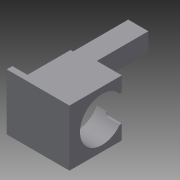
# Autodesk Inventor part: BF_base_model
Saved by Autodesk Inventor 2015 SP2 (Build 190223200, 223)
## iProperties
Created: 2016-08-30
Part Number: BF_base_model
Material: Generic
Document SubType Name: Modeling
Designer: jm799
Density: 1 g/cm^3
Appearance: Default
Author: jm799
Autodesk Inventor part; units mm, degrees
ref_plane "YZ Plane" through (0, 0, 0) normal (1, 0, 0) x (0, 1, 0)
ref_plane "XZ Plane" through (0, 0, 0) normal (0, 1, 0) x (-1, 0, 0)
ref_plane "XY Plane" through (0, 0, 0) normal (0, 0, 1) x (1, 0, 0)
sketch "Sketch1" plane through (0, 0, 0) normal (0, 1, 0) x (-1, 0, 0)
  line L0 (16.2222, 35.2121) -> (-14.7778, 35.2121)
  line L1 (-14.7778, 35.2121) -> (-14.7778, -34.7879)
  line L2 (-14.7778, -34.7879) -> (16.2222, -34.7879)
  line L3 (16.2222, -34.7879) -> (16.2222, 35.2121)
  point P0 (0, 0)
  dimension "d0" = 70
  dimension "d1" = 31
  constraints: 8 end point, 2 parallel, 1 horizontal, 1 perpendicular
  measures "d0" distance of L0.end L1.end
  measures "d1" distance of L0.start L0.end
extrude "Extrusion1" add sketch "Sketch1" along normal blind 60
sketch "Sketch3" plane through (14.7778, 0, 35.2121) normal (1, 0, 0) x (0, 0, -1)
  circle A0 centre (35.2121, 35.5368) radius 27.5
  point P0 (35.2121, 0)
  dimension "d5" = 55
  constraints: 1 centre point
  measures "d5" diameter of A0
hole "Hole1" at (14.7778, 35.5368, 0) direction (-1, 0, 0) diameter 55 end through all
sketch "Sketch6" plane through (0, 60, 0) normal (0, 1, 0) x (1, 0, 0)
  line L0 (-0.0667, -13.4045) -> (-0.0667, 12.7365)
  line L1 (-16.2222, 0) -> (14.7778, 0) construction
  circle A0 centre (-0.0667, -12.8895) radius 4
  circle A1 centre (-0.0667, 12.5336) radius 4
  point P0 (0, 0)
  point P1 (14.7778, -12.562)
  point P2 (-16.2222, -12.562)
  point P3 (-16.2222, 12.562)
  point P4 (14.7778, 12.562)
  dimension "d42" = 8
  dimension "d43" = 8
  constraints: 4 end point, 2 centre point, 1 vertical
  measures "d42" diameter of A0
  measures "d43" diameter of A1
sketch "Sketch8" plane through (0, 60, 0) normal (0, 1, 0) x (1, 0, 0)
  line L0 (14.7778, 34.7879) -> (-16.2222, 34.7879) construction
  line L1 (-16.2222, 0) -> (14.7778, 0) construction
  circle A0 centre (5, -28) radius 2
  circle A1 centre (5, 28) radius 2
  point P0 (0, 0)
  dimension "d33" = 4
  constraints: 2 centre point, 2 end point, 1 horizontal, 1 symmetric about line, 1 other
  measures "d33" diameter of A0
extrude "Extrusion4" cut sketch "Sketch6" against normal blind 4
sketch "Sketch15" plane through (0, 60, 0) normal (0, 1, 0) x (1, 0, 0)
  arc A0 (-4.0532, -12.562) -> (3.9199, -12.562) centre (-0.0667, -12.8895) ccw projected
  line L0 (-0.0667, -16.8895) -> (14.7778, -16.8895)
  line L1 (14.7778, 27.5) -> (14.7778, -27.5) projected
  line L2 (14.7778, -12.562) -> (14.7778, -16.8895)
  line L3 (14.7778, -12.562) -> (3.9199, -12.562) projected
  line L4 (-0.0667, -12.8895) -> (-0.0667, -12.8895)
  arc A1 (3.9332, 12.562) -> (-4.0666, 12.562) centre (-0.0667, 12.5336) ccw projected
  line L5 (-0.0667, 16.5336) -> (-0.0667, 12.5336)
  line L6 (3.9332, 12.562) -> (14.7778, 12.562) projected
  line L7 (14.7778, 12.562) -> (14.7778, 16.5336)
  line L8 (14.7778, 16.5336) -> (-0.0667, 16.5336)
  line L9 (-0.0667, -12.562) -> (14.7778, -12.562)
  line L10 (-0.0667, -12.562) -> (-0.0667, -16.8895)
  line L11 (14.7778, 12.562) -> (-0.0667, 12.5336)
  point P0 (0, 0)
  constraints: 18 end point, 2 collinear, 2 perpendicular, 2 point on circle, 2 point on line, 2 tangent, 1 horizontal, 1 vertical
extrude "Extrusion5" cut sketch "Sketch15" against normal blind 4 contours A0 L3 L1 L0 | L1 L6 A1 L8
hole "Hole5" at (5, 60, 28) at (5, 60, -28) direction (0, -1, 0) diameter 5 depth 14
sketch "Sketch18" plane through (0, 0, 0) normal (0, -1, 0) x (1, 0, 0)
  line L0 (-16.2222, -34.7879) -> (-63.2222, -34.7879)
  line L1 (-16.2222, 35.2121) -> (-63.2222, 35.2121)
  line L2 (-63.2222, 35.2121) -> (-63.2222, -34.7879)
  line L3 (-16.2222, -34.7879) -> (-16.2222, 35.2121)
  line L4 (-63.2222, -34.7879) -> (-63.2222, 35.2121)
  point P0 (0, 0)
  dimension "d57" = 47
  constraints: 10 end point, 2 horizontal, 1 collinear, 1 perpendicular, 1 vertical
  measures "d57" distance of L0.start L0.end
extrude "Extrusion9" add sketch "Sketch18" against normal blind 2
sketch "Sketch25" plane through (0, 0, 0) normal (0, -1, 0) x (1, 0, 0)
  line L0 (-63.2222, 35.2121) -> (14.7778, 35.2121)
  line L1 (14.7778, 35.2121) -> (14.7778, -34.7879)
  line L2 (14.7778, -34.7879) -> (-63.2222, -34.7879)
  line L3 (-63.2222, -34.7879) -> (-63.2222, 35.2121)
  point P0 (0, 0)
  constraints: 8 end point, 2 parallel, 1 horizontal, 1 perpendicular
extrude "Extrusion11" add sketch "Sketch25" along normal blind 5
sketch "Sketch29" plane through (0, 2, 0) normal (0, 1, 0) x (1, 0, 0)
  point P0 (0, 0)
sketch "Sketch37" plane through (0, 2, 0) normal (0, 1, 0) x (1, 0, 0)
  point P0 (0, 0)
sketch "Sketch39" plane through (0, 2, 0) normal (0, 1, 0) x (1, 0, 0)
  line L0 (-16.2222, -35.2121) -> (-41.2222, -35.2121)
  line L1 (-41.2222, -35.2121) -> (-41.2222, -12.2121)
  line L2 (-41.2222, -12.2121) -> (-16.2222, -12.2121)
  line L3 (-16.2222, -12.2121) -> (-16.2222, -35.2121)
  point P0 (0, 0)
  dimension "d120" = 25
  dimension "d121" = 23
  constraints: 8 end point, 2 parallel, 1 horizontal, 1 perpendicular
  measures "d120" distance of L1.end L2.end
  measures "d121" distance of L0.end L1.end
extrude "Extrusion27" add sketch "Sketch39" along normal blind 122
sketch "Sketch43" plane through (0, 2, 0) normal (0, 1, 0) x (1, 0, 0)
  line L0 (-16.2222, 34.7879) -> (-63.2222, 34.7879) projected
  line L1 (-41.2222, -35.2121) -> (-44.39, -35.2121)
  line L2 (-44.39, -35.2121) -> (-44.39, 34.7879)
  line L3 (-44.39, 34.7879) -> (-41.2222, 34.7879)
  line L4 (-41.2222, 34.7879) -> (-41.2222, -35.2121)
  point P0 (0, 0)
  constraints: 8 end point, 2 parallel, 1 horizontal, 1 perpendicular, 1 point on line
extrude "Extrusion28" add sketch "Sketch43" along normal blind 53.526
body "Solid1"
